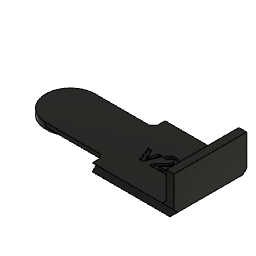
Connector_Lid_M2 (Autodesk Fusion 360 design; units mm, degrees)
Autodesk Fusion 360 part; units mm, degrees
sketch "Skizze1" plane through (0, 0, 0) normal (1, 0, 0) x (0, 1, 0)
  line L0 (9.5, -1) -> (-9.5, -1) construction
  line L1 (-9.5, -1) -> (-9.5, 1) construction
  line L2 (-9.5, 1) -> (9.5, 1) construction
  line L3 (9.5, 1) -> (9.5, -1) construction
  line L4 (9.5, -1) -> (-9.5, 1) construction
  line L5 (-9.5, -1) -> (9.5, 1) construction
  line L6 (-9.5, 1) -> (-8.5, 0) construction
  line L7 (-8.5, 0) -> (-9.5, -1) construction
  line L8 (9.5, 1) -> (8.5, 0) construction
  line L9 (8.5, 0) -> (9.5, -1) construction
  line L10 (-9.35, 1) -> (-8.35, 0)
  line L11 (-8.35, 0) -> (-9.35, -1)
  line L12 (9.35, 1) -> (8.35, 0)
  line L13 (8.35, 0) -> (9.35, -1)
  line L14 (-9.35, 1) -> (9.35, 1)
  line L15 (9.35, -1) -> (-9.35, -1)
  dimension "d103" = 2
  dimension "d104" = 135
  dimension "d105" = 135
  dimension "d110" = 19
  dimension "d129" = 0.15
  dimension "d130" = 0.15
  constraint horizontal L0
  constraint perpendicular L0 L1
  constraint parallel L0 L2
  constraint parallel L1 L3
  constraint coincident L4 origin
  constraint coincident L5 origin
  constraint horizontal origin L6.end
  constraint horizontal origin L8.end
  constraint coincident L2 L10.start
  constraint coincident L0 L11.end
  constraint parallel L6 L10
  constraint parallel L7 L11
  constraint horizontal origin L10.end
  constraint coincident L2 L12.start
  constraint coincident L0 L13.end
  constraint parallel L8 L12
  constraint parallel L9 L13
  constraint horizontal origin L12.end
  measures "d103" distance of L0.end L1.end
  measures "d104" angle of L1 L6
  measures "d105" angle of L3 L8
  measures "d110" distance of L1 L3
  measures "d129" distance of L6.end L10.end
  measures "d130" distance of L8.end L12.end
extrude "Extrusion1" add sketch "Skizze1" along normal blind 21
sketch "Skizze2" plane through (21, 0, 0) normal (1, 0, 0) x (0, 1, 0)
  line L0 (-9.35, 1) -> (-8.35, 0)
  line L1 (-8.35, 0) -> (-9.35, -1)
  line L2 (-9.35, -1) -> (9.35, -1)
  line L3 (9.35, -1) -> (8.35, 0)
  line L4 (8.35, 0) -> (9.35, 1)
  line L5 (9.35, 1) -> (-9.35, 1)
  line L6 (-9.35, 1) -> (9.35, 1)
  line L7 (9.35, 1) -> (9.35, 9)
  line L8 (9.35, 9) -> (-9.35, 9)
  line L9 (-9.35, 9) -> (-9.35, 1)
  dimension "d111" = 8
  constraint horizontal L6
  constraint vertical L7
  constraint horizontal L8
  constraint vertical L9
  constraint coincident L0.start L5.end
  constraint coincident L4.end L5.start
  measures "d111" distance of L4.end L7.end
extrude "Extrusion2" add sketch "Skizze2" against normal blind 2 contours L5 L6 L7 L8 L9
sketch "Skizze3" plane through (0, 0, 1) normal (0, 0, 1) x (-1, 0, 0)
  line L0 (-19, 9.35) -> (-19, -9.35)
  line L1 (-19, -9.35) -> (0, -9.35)
  line L2 (0, -9.35) -> (0, 9.35)
  line L3 (0, 9.35) -> (-19, 9.35)
  circle A0 centre (15, 0) radius 6.5 construction
  line L4 (15, -6.5) -> (0, -6.5) construction
  line L5 (15, 6.5) -> (0, 6.5) construction
  line L6 (0, -6.35) -> (15, -6.35)
  line L7 (0, 6.35) -> (15, 6.35)
  circle A1 centre (15, 0) radius 6.35
  line L8 (0, -6.35) -> (0, 6.35)
  dimension "d114" = 13
  dimension "d115" = 15
  dimension "d116" = 0.15
  dimension "d117" = 0.15
  constraint coincident A0 L4.start
  constraint coincident L2 L4.end
  constraint perpendicular L2 L4
  constraint coincident A0 L5.start
  constraint coincident L2 L5.end
  constraint perpendicular L2 L5
  constraint tangent A0 L4
  constraint tangent A0 L5
  constraint horizontal origin A0.centre
  constraint coincident L2 L6.start
  constraint perpendicular L2 L6
  constraint coincident L2 L7.start
  constraint perpendicular L2 L7
  constraint concentric A0 A1
  constraint coincident L7.end A1
  constraint tangent L6 A1
  constraint coincident A1 L6.end
  measures "d114" diameter of A0
  measures "d115" distance of L5.start L5.end
  measures "d116" distance of L4 L6
  measures "d117" distance of L5 L7
extrude "Extrusion3" add sketch "Skizze3" against normal blind 1 contours L2 L6 L7 A1 L8 | A1
extrude "Extrusion4" add sketch "Skizze3" against normal blind 1 from surface at -1 contours A1
chamfer "Fase1" distance 0.5 angle 45 1 edges at (-9.0797, -2.2963, -1)
chamfer "Fase1" distance 1 angle 45 4 edges at (0, -6.35, 0.5) (0, 6.35, 0.5) (19, 0, 1) (21, 0, -1)
sketch "Skizze4" plane through (0, 0, 0) normal (0, 1, 0) x (1, 0, 0)
  line L0 (-21.35, -1) -> (-15, -1)
  line L1 (-15, -1) -> (-15, 0)
  line L2 (-15, 0) -> (-8.65, 0)
  line L3 (-15, 0) -> (-15, -1)
  line L4 (-8.65, 0.5) -> (-21.35, 0.5)
  line L5 (-8.65, 0.5) -> (-21.35, 0.5)
  line L6 (-20.85, 1) -> (-9.15, 1)
  line L7 (-21.35, -0.25) -> (-19.1849, 1)
  line L8 (-21.35, -0.25) -> (-17.5, -0.25) construction
  line L9 (-21.35, -0.25) -> (-21.35, 0.5)
  line L10 (-21.35, 0.5) -> (-20.85, 1)
  line L11 (-19.1849, 1) -> (-20.85, 1)
  line L12 (-8.65, 0) -> (-10.3821, 1)
  line L13 (-9.15, 1) -> (-8.65, 0.5)
  line L14 (-8.65, 0) -> (-8.65, 0.5)
  dimension "d126" = 30
  dimension "d127" = 0.75
  dimension "d437" = 30
  constraint horizontal L8
  constraint coincident L6 L7.end
  constraint vertical L0.start L7.start
  constraint coincident L4.end L5.end
  constraint coincident L6.start L10.end
  constraint coincident L2.end L12.start
  constraint coincident L6 L12.end
  constraint coincident L6.end L13.start
  constraint coincident L4.start L5.start
  measures "d126" angle of L7 L8
  measures "d127" distance of L0.start L7.start
  measures "d437" angle of L2 L12
extrude "Extrusion5" cut sketch "Skizze4" along normal through all and the other way through all contours L4 L5 L12 L14 | L4 L5 L6 L12 L13 | L4 L5 L7 L9 | L4 L5 L6 L7 L10 L11
sketch "Skizze5" plane through (0, 0, -1) normal (0, 0, -1) x (1, 0, 0)
  line L0 (20, -9.35) -> (20, 9.35)
  line L1 (20, 9.35) -> (0, 9.35)
  line L2 (0, 9.35) -> (0, -9.35)
  line L3 (0, -9.35) -> (20, -9.35)
  line L4 (18, 0) -> (3, 6.35) construction
  line L5 (3, 6.35) -> (3, -6.35)
  line L6 (3, -6.35) -> (18, 0) construction
  line L7 (5, -5.5033) -> (5, 5.5033)
  line L8 (9.5, 3.5983) -> (9.5, -3.5983)
  line L9 (11.5, -2.7517) -> (11.5, 2.7517)
  line L10 (16, 0.8467) -> (16, -0.8467)
  line L11 (16, 0.8467) -> (18, 0)
  line L12 (18, 0) -> (16, -0.8467)
  line L13 (5, 0) -> (9.5, 0) construction
  line L14 (11.5, 0) -> (16, 0) construction
  line L15 (3, 6.35) -> (5, 5.5033)
  line L16 (9.5, 3.5983) -> (11.5, 2.7517)
  line L17 (11.5, -2.7517) -> (9.5, -3.5983)
  line L18 (5, -5.5033) -> (3, -6.35)
  dimension "d138" = 3
  dimension "d139" = 2
  dimension "d140" = 3
  dimension "d141" = 2
  dimension "d142" = 2
  dimension "d143" = 2
  constraint parallel L0 L5
  constraint equal L4 L6
  constraint horizontal origin L4.start
  constraint coincident L6 L7.start
  constraint coincident L4 L7.end
  constraint parallel L2 L7
  constraint coincident L4 L8.start
  constraint coincident L6 L8.end
  constraint parallel L7 L8
  constraint coincident L6 L9.start
  constraint coincident L4 L9.end
  constraint parallel L7 L9
  constraint coincident L4 L10.start
  constraint coincident L6 L10.end
  constraint parallel L9 L10
  constraint midpoint L7 L13.start
  constraint midpoint L8 L13.end
  constraint midpoint L9 L14.start
  constraint midpoint L10 L14.end
  constraint equal L13 L14
  measures "d138" distance of L2 L5
  measures "d139" distance of L0 L4.start
  measures "d140" distance of L1 L4.end
  measures "d141" distance of L4.start L10
  measures "d142" distance of L8 L9
  measures "d143" distance of L5 L7
extrude "Extrusion6" cut sketch "Skizze5" against normal blind 0.5 contours L5 L7 L15 L18 | L8 L9 L16 L17 | L10 L11 L12
sketch "Skizze7" plane through (0, 0, 1) normal (0, 0, 1) x (-1, 0, 0)
  line L0 (-18, 9.35) -> (-18, -9.35)
  line L1 (-18, -9.35) -> (0, -9.35)
  line L2 (0, -9.35) -> (0, -7.35)
  line L3 (0, -7.35) -> (1, -6.35)
  line L4 (1, -6.35) -> (15, -6.35)
  arc A0 (15, -6.35) -> (15, 6.35) centre (15, 0) ccw
  line L5 (15, 6.35) -> (1, 6.35)
  line L6 (1, 6.35) -> (0, 7.35)
  line L7 (0, 7.35) -> (0, 9.35)
  line L8 (0, 9.35) -> (-18, 9.35)
  line L9 (-4, 2.5) -> (-15, 2.5) construction
  line L10 (-15, 2.5) -> (-15, -2.5) construction
  line L11 (-15, -2.5) -> (-4, -2.5) construction
  line L12 (-4, -2.5) -> (-4, 2.5) construction
  dimension "d363" = 5
  dimension "d364" = 5
  dimension "d365" = 11
  dimension "d366" = 3
  text T0 "v22" font "Arial" height 5 bold align centre middle in box 11 x 5 at (-4, 2.5) x (-1, 0) y (0, -1) spacing 1
  constraint horizontal origin
  measures "d366" distance of L0 L10
extrude "Extrusion7" cut sketch "Skizze7" against normal blind 0.5 text T0
equation "d108 = 17 mm + 4 mm"
equation "d117 = d116"
equation "d130 = d129"
equation "d142 = d141"
equation "d143 = d141"
named bodies: "Connector_Lid"
